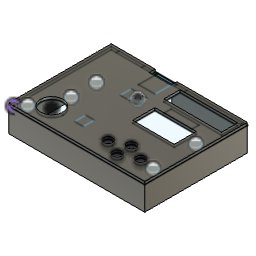
SmartDiskII Case v18 (Autodesk Fusion 360 design; units mm, degrees)
Autodesk Fusion 360 part; units mm, degrees
note: some values were not read from the file. Chosen so that the rebuilt part matches the saved one: which bodies a step acts on; which face or edge a step refers to. Set by a fixed rule: which sketch regions a step uses.
sketch "Sketch1" plane through (0, 0, 0) normal (0, 0, 1) x (1, 0, 0)
  line L0 (0, 0) -> (76.3, 0)
  line L1 (76.3, 0) -> (76.3, 56.8)
  line L2 (76.3, 56.8) -> (0, 56.8)
  line L3 (0, 56.8) -> (0, 0)
  line L4 (77.8, 58.3) -> (-1.5, 58.3)
  line L5 (-1.5, 58.3) -> (-1.5, -1.5)
  line L6 (-1.5, -1.5) -> (77.8, -1.5)
  line L7 (77.8, -1.5) -> (77.8, 58.3)
  line L8 (2.9, 56.8) -> (2.9, 58.3)
  line L9 (17.8, 56.8) -> (17.8, 58.3)
  line L10 (25.6, 56.8) -> (25.6, 58.3)
  line L11 (35.2, 58.3) -> (35.2, 56.8)
  line L12 (75.3, 58.3) -> (75.3, 56.8)
  line L13 (42.6, 58.3) -> (42.6, 56.8)
  line L14 (43.4, 38.8) -> (67.6, 38.8)
  line L15 (67.6, 38.8) -> (67.6, 25.9)
  line L16 (67.6, 25.9) -> (43.4, 25.9)
  line L17 (43.4, 25.9) -> (43.4, 38.8)
  circle A0 centre (65.2, 8.8) radius 2.5
  circle A1 centre (46.2, 8.8) radius 2.5
  circle A2 centre (55.6, 4.6) radius 2.5
  circle A3 centre (55.6, 12.9) radius 2.5
  line L18 (41.7, 55.2) -> (75.3, 55.2)
  line L19 (75.3, 55.2) -> (75.3, 45.8)
  line L20 (75.3, 45.8) -> (41.7, 45.8)
  line L21 (41.7, 45.8) -> (41.7, 55.2)
  line L22 (25.6, 56.8) -> (35.2, 56.8)
  line L23 (35.2, 56.8) -> (35.2, 47.1)
  line L24 (35.2, 47.1) -> (25.6, 47.1)
  line L25 (25.6, 47.1) -> (25.6, 56.8)
  line L26 (25.6, 42.9) -> (35.2, 42.9)
  line L27 (35.2, 42.9) -> (35.2, 36.4)
  line L28 (35.2, 36.4) -> (25.6, 36.4)
  line L29 (25.6, 36.4) -> (25.6, 42.9)
  circle A4 centre (12.4, 9.7) radius 6.5
  line L30 (25.6, 16.35) -> (30.6, 16.35)
  line L31 (30.6, 16.35) -> (30.6, 9.85)
  line L32 (30.6, 9.85) -> (25.6, 9.85)
  line L33 (25.6, 9.85) -> (25.6, 16.35)
  circle A5 centre (12.4, 21) radius 2.5
  circle A6 centre (12.4, 35.8) radius 2.5
  circle A7 centre (72.3819, 33.8) radius 2.5
  circle A8 centre (3.8963, 4.2747) radius 2.5
  circle A9 centre (72.3819, 8.8) radius 2.5
  line L34 (47.4, 40.3) -> (63.6, 40.3)
  line L35 (63.6, 40.3) -> (63.6, 44.3)
  line L36 (63.6, 44.3) -> (47.4, 44.3)
  line L37 (47.4, 44.3) -> (47.4, 40.3)
  line L38 (24.1, 58.3) -> (36.7, 58.3)
  line L39 (36.7, 58.3) -> (36.7, 56.8)
  line L40 (36.7, 56.8) -> (24.1, 56.8)
  line L41 (24.1, 56.8) -> (24.1, 58.3)
  line L42 (30.1, 42.9) -> (30.1, 36.4)
  line L43 (30.1, 36.4) -> (35.2, 42.9) construction
  line L44 (30.1, 42.9) -> (35.2, 36.4) construction
  circle A10 centre (32.65, 39.65) radius 2
  dimension "d5" = 76.3
  dimension "d6" = 56.8
  dimension "d8" = 1.5
  dimension "d9" = 2.9
  dimension "d10" = 17.8
  dimension "d11" = 25.6
  dimension "d12" = 35.2
  dimension "d13" = 75.3
  dimension "d14" = 42.6
  dimension "d15" = 8.7
  dimension "d16" = 24.2
  dimension "d17" = 12.9
  dimension "d18" = 25.9
  dimension "d19" = 5
  dimension "d20" = 8.8
  dimension "d21" = 11.1
  dimension "d22" = 5
  dimension "d23" = 30.1
  dimension "d24" = 5
  dimension "d25" = 4.6
  dimension "d26" = 20.7
  dimension "d27" = 5
  dimension "d28" = 12.9
  dimension "d39" = 9.4
  dimension "d40" = 1.6
  dimension "d43" = 8.8
  dimension "d44" = 1
  dimension "d45" = 33.6
  dimension "d46" = 20.7
  dimension "d47" = 9.7
  dimension "d48" = 6.5
  dimension "d50" = 13.9
  dimension "d53" = 13
  dimension "d54" = 12.4
  dimension "d55" = 9.7
  dimension "d58" = 9.85
  dimension "d59" = 6.5
  dimension "d60" = 5
  dimension "d67" = 5
  dimension "d68" = 5
  dimension "d69" = 21
  dimension "d70" = 21
  dimension "d71" = 5
  dimension "d72" = 5
  dimension "d73" = 23
  dimension "d74" = 5
  dimension "d86" = 4
  dimension "d87" = 4
  dimension "d88" = 1.5
  dimension "d89" = 1.5
  dimension "d92" = 12.6
  dimension "d93" = 1.5
  dimension "d94" = 1.5
  dimension "d113" = 4.5
  dimension "d135" = 4
  constraint horizontal L0
  constraint vertical L1
  constraint horizontal L2
  constraint vertical L3
  constraint coincident L0.start L3.end
  constraint coincident L2 L8.start
  constraint coincident L4 L8.end
  constraint perpendicular L4 L8
  constraint coincident L2 L9.start
  constraint coincident L4 L9.end
  constraint perpendicular L4 L9
  constraint coincident L2 L10.start
  constraint coincident L4 L10.end
  constraint perpendicular L4 L10
  constraint coincident L4 L11.start
  constraint coincident L2 L11.end
  constraint perpendicular L2 L11
  constraint coincident L4 L12.start
  constraint coincident L2 L12.end
  constraint perpendicular L2 L12
  constraint coincident L4 L13.start
  constraint coincident L2 L13.end
  constraint perpendicular L2 L13
  constraint horizontal L14
  constraint vertical L15
  constraint horizontal L16
  constraint vertical L17
  constraint horizontal L18
  constraint vertical L19
  constraint horizontal L20
  constraint vertical L21
  constraint horizontal L22
  constraint vertical L23
  constraint horizontal L24
  constraint vertical L25
  constraint horizontal L26
  constraint vertical L27
  constraint horizontal L28
  constraint vertical L29
  constraint horizontal L30
  constraint vertical L31
  constraint horizontal L32
  constraint vertical L33
  constraint collinear L29 L33
  constraint horizontal L34
  constraint vertical L35
  constraint horizontal L36
  constraint vertical L37
  constraint horizontal L38
  constraint vertical L39
  constraint horizontal L40
  constraint vertical L41
  constraint coincident L4 L38.start
  constraint coincident L26 L42.start
  constraint coincident L28 L42.end
  constraint perpendicular L28 L42
  constraint midpoint L44 A10.centre
  measures "d5" distance of L0.start L0.end
  measures "d6" distance of L0.start L2.end
  measures "d9" distance of L3 L8
  measures "d10" distance of L3 L9
  measures "d11" distance of L3 L10
  measures "d12" distance of L3 L11
  measures "d13" distance of L3 L12
  measures "d14" distance of L3 L13
  measures "d15" distance of L1 L15
  measures "d16" distance of L15 L17
  measures "d17" distance of L14 L16
  measures "d18" distance of L0 L16
  measures "d19" diameter of A0
  measures "d20" distance of L0 A0.centre
  measures "d21" distance of L1 A0.centre
  measures "d22" diameter of A1
  measures "d23" distance of L1 A1.centre
  measures "d24" diameter of A2
  measures "d25" distance of L0 A2.centre
  measures "d26" distance of L1 A2.centre
  measures "d27" diameter of A3
  measures "d28" distance of L0 A3.centre
  measures "d39" distance of L18.start L20.end
  measures "d40" distance of L2 L18
  measures "d43" distance of L0 A1.centre
  measures "d44" distance of L1 L19
  measures "d45" distance of L19 L21
  measures "d46" distance of L1 A3.centre
  measures "d47" distance of L10.start L24.end
  measures "d48" distance of L26.start L28.end
  measures "d50" distance of L2 L26
  measures "d53" diameter of A4
  measures "d54" distance of L3 A4.centre
  measures "d55" distance of L0 A4.centre
  measures "d58" distance of L0 L32
  measures "d59" distance of L30 L32
  measures "d60" distance of L31 L33
  measures "d67" diameter of A5
  measures "d68" diameter of A6
  measures "d69" distance of L2 A6.centre
  measures "d70" distance of L0 A5.centre
  measures "d71" diameter of A7
  measures "d72" diameter of A8
  measures "d73" distance of L2 A7.centre
  measures "d74" diameter of A9
  measures "d86" distance of L17 L37
  measures "d87" distance of L15 L35
  measures "d88" distance of L20 L36
  measures "d89" distance of L14 L34
  measures "d92" distance of L38.start L38.end
  measures "d93" distance of L10 L41
  measures "d94" distance of L11 L39
  measures "d113" distance of L29 L42
  measures "d135" diameter of A10
extrude "Extrude1" add sketch "Sketch1" along normal blind 1.5 contours L0 L1 L2 L3 L23 L24 L25 L40 | L2 L22 L23 L24 L25 L40 | L18 L19 L20 L21 | L26 L28 L29 L42 | L26 L27 L28 L42 | A4 | L30 L31 L32 L33 | A5 | A6 | A7 | A8 | A9 | L34 L35 L36 L37 | A10 makes body 1
extrude "Extrude2" add sketch "Sketch1" against normal blind 10 contours L0 L1 L2 L3 L4 L5 L6 L7 L8 L12 | L2 L4 L12 L13 | L2 L4 L9 L41 | L2 L4 L13 L39 | L2 L4 L10 L38 L40 L41 | L2 L4 L11 L38 L39 L40 bodies 1
extrude "Extrude3" add sketch "Sketch1" along normal blind 1.5 separate body contours L0 L1 L2 L3 L4 L5 L6 L7 L8 L12 | L2 L4 L8 L9 | L2 L4 L12 L13 | L2 L4 L9 L41 | L2 L4 L13 L39 | L2 L4 L10 L38 L40 L41 | L2 L4 L11 L38 L39 L40 | L2 L4 L10 L11 L22 L38 L40 makes body 2
extrude "Extrude4" cut sketch "Sketch1" along normal blind 1.5 contours L18 L19 L20 L21 bodies 1
extrude "Extrude5" cut sketch "Sketch1" along normal blind 3 contours L2 L4 L10 L11 L22 L38 L40 | L2 L22 L23 L24 L25 L40 | L26 L28 L29 L42 | L26 L27 L28 L42 | A4 | L30 L31 L32 L33 | A10 bodies 1 2
sketch "Sketch2" plane through (0, 0, 0) normal (0, 0, 1) x (1, 0, 0)
  circle A0 centre (55.6, 12.9) radius 2.25
  circle A1 centre (55.6, 12.9) radius 3.25
  line L0 (1.5, 1.5) -> (74.8, 1.5)
  line L1 (74.8, 1.5) -> (74.8, 55.3)
  line L2 (74.8, 55.3) -> (1.5, 55.3)
  line L3 (1.5, 55.3) -> (1.5, 1.5)
  line L4 (0, 56.8) -> (0, 0)
  line L5 (0, 0) -> (76.3, 0)
  line L6 (76.3, 0) -> (76.3, 56.8)
  line L7 (76.3, 56.8) -> (0, 56.8)
  line L8 (76.2, 0.1) -> (0.1, 0.1)
  line L9 (0.1, 0.1) -> (0.1, 56.7)
  line L10 (0.1, 56.7) -> (76.2, 56.7)
  line L11 (76.2, 56.7) -> (76.2, 0.1)
  circle A2 centre (32.65, 39.65) radius 2.5
  circle A3 centre (32.65, 39.65) radius 1.75
  point P0 (55.6, 12.9)
  point P1 (32.65, 39.65)
  dimension "d61" = 4.5
  dimension "d62" = 6.5
  dimension "d101" = 1.5
  dimension "d102" = 1.5
  dimension "d103" = 1.5
  dimension "d104" = 1.5
  dimension "d121" = 0.1
  dimension "d122" = 0.1
  dimension "d123" = 0.1
  dimension "d124" = 0.1
  dimension "d136" = 5
  dimension "d137" = 3.5
  constraint coincident P0 A0.centre
  constraint horizontal L0
  constraint vertical L1
  constraint horizontal L2
  constraint vertical L3
  constraint horizontal L8
  constraint vertical L9
  constraint horizontal L10
  constraint vertical L11
  constraint coincident P1 A2.centre
  constraint concentric A2 A3
  measures "d61" diameter of A0
  measures "d62" diameter of A1
  measures "d101" distance of L3 L4
  measures "d102" distance of L0 L5
  measures "d103" distance of L1 L6
  measures "d104" distance of L2 L7
  measures "d121" distance of L7 L10
  measures "d122" distance of L6 L11
  measures "d123" distance of L5 L8
  measures "d124" distance of L4 L9
  measures "d136" diameter of A2
  measures "d137" diameter of A3
extrude "Extrude7" add sketch "Sketch2" along normal blind 1.7 separate body contours A1 makes body 3
extrude "Extrude8" add sketch "Sketch2" along normal blind 4 contours A0 bodies 3
extrude "Extrude9" add sketch "Sketch1" against normal blind 6.9 separate body contours A5 | A6 | A7 | A8 | A9 makes body 4 at (6.3932, 4.15, -4.6) makes body 5 at (14.8969, 35.6754, -4.6) makes body 6 at (74.8788, 33.6754, -4.6) makes body 7 at (14.8969, 20.8754, -4.6) makes body 8 at (74.8788, 8.6754, -4.6)
combine "Combine1" operation add target body 4 tool bodies 7 5 6 8 makes body 9 at (14.8969, 20.8754, -4.6) makes body 10 at (74.8788, 33.6754, -4.6) makes body 11 at (14.8969, 35.6754, -4.6) makes body 12 at (74.8788, 8.6754, -4.6)
extrude "Extrude10" add sketch "Sketch1" against normal blind 5 contours L2 L4 L8 L9 bodies 1 3 2
extrude "Extrude11" add 2 faces at (25.4333, -1, -10) (23, 57.3, -10) along direction (0, 0, -1) blind 4 on bodies 1 bodies 1
extrude "Extrude12" add sketch "Sketch1" along normal blind 0.75 from surface at 0.75 contours L2 L22 L23 L24 L25 L40 | L30 L31 L32 L33 bodies 1
extrude "Extrude13" cut 1 faces at (32, 56.8, 1) along direction (0, -1, 0) blind 2 on bodies 1 bodies 1
extrude "Extrude14" cut sketch "Sketch1" along normal blind 0.75 contours L34 L35 L36 L37 bodies 1
extrude "Extrude15" cut sketch "Sketch1" along normal blind 1.5 contours L2 L4 L10 L38 L40 L41 | L2 L4 L11 L38 L39 L40 bodies 1
extrude "Extrude16" cut 2 faces at (36.2, 56.8, 0.5) (25.1, 56.8, 1) along direction (0, 1, 0) up to surface end surface through (35.2, 54.8, 0.75) normal (0, 1, 0) offset 0 on bodies 1 bodies 1
extrude "Extrude17" cut sketch "Sketch1" against normal blind 4 contours L2 L4 L10 L38 L40 L41 | L2 L4 L11 L38 L39 L40 bodies 1
fillet "Fillet1" radius 2 1 edges at (24.1, 57.55, -4) on bodies 1
fillet "Fillet1" radius 2 1 edges at (36.7, 57.55, -4) on bodies 1
extrude "Extrude18" add sketch "Sketch1" sketch "Sketch2" along normal blind 1.5 separate body contours L0 L1 L2 L3 L4 L5 L6 L7 L8 L12 | L2 L4 L8 L9 | L2 L4 L12 L13 | L2 L4 L9 L41 | L2 L4 L13 L39 | L2 L4 L10 L38 L40 L41 | L2 L4 L11 L38 L39 L40 | L2 L4 L10 L11 L22 L38 L40 of sketch 2 contours A0 | A1 | L0 L1 L2 L3 | L4 L5 L6 L7 | L8 L9 L10 L11 | A2 | A3 makes body 13
extrude "Extrude19" add sketch "Sketch2" along normal blind 6.7 contours L8 L9 L10 L11 bodies 13
extrude "Extrude20" add sketch "Sketch1" along normal blind 8.6 contours L2 L4 L8 L9 bodies 13
extrude "Extrude21" add sketch "Sketch1" along normal blind 9.5 contours L2 L4 L10 L11 L22 L38 L40 bodies 13
extrude "Extrude22" add sketch "Sketch1" along normal blind 0.75 from surface at 0.75 contours L26 L28 L29 L42 bodies 1
extrude "Extrude23" add 1 faces at (28.8, 57.8, 9.5) along direction (0, 0, 1) blind 2 on bodies 13 bodies 13
extrude "Extrude24" cut 1 faces at (25.6, 57.8, 8.1667) along direction (1, 0, 0) blind 0.1 on bodies 13 bodies 13
extrude "Extrude25" cut 1 faces at (2.9, 57.8, 6.2333) along direction (1, 0, 0) blind 0.1 on bodies 13 bodies 13
extrude "Extrude26" cut 1 faces at (17.8, 57.8, 6.2333) along direction (-1, 0, 0) blind 0.1 on bodies 13 bodies 13
extrude "Extrude27" cut 1 faces at (35.2, 57.8, 4.8333) along direction (-1, 0, 0) blind 0.1 on bodies 13 bodies 13
extrude "Extrude28" add sketch "Sketch2" along normal blind 0.5 separate body contours A2 makes body 14
extrude "Extrude29" add sketch "Sketch2" along normal blind 1.75 contours A3 bodies 14
extrude "Extrude30" add sketch "Sketch1" along normal blind 0.75 from surface at 0.75 contours L26 L27 L28 L42 bodies 1
hidden bodies 3 4 9 10 11 12 13 14
equation "width = 76 mm"
equation "length = 56.5 mm"
equation "margin = 0.3 mm"
equation "d5 = width + margin"
equation "d6 = length + margin"
equation "wall_ep = 1.5 mm"
equation "d8 = wall_ep"
equation "d9 = margin + 2.6 mm"
equation "d10 = margin + 17.5 mm"
equation "d11 = margin + 25.3 mm"
equation "d12 = margin + 34.90 mm"
equation "d13 = margin + 75 mm"
equation "d14 = margin + 42.30 mm"
equation "d33 = wall_ep"
equation "d37 = wall_ep"
equation "d39 = 8.8 mm + 0.6 mm"
equation "d40 = 1.9 mm - 0.3 mm"
equation "d41 = wall_ep"
equation "d45 = 33.10 mm + 0.5 mm"
equation "d77 = -5.6 mm + 1.5 mm - 0.9 mm"
equation "d101 = wall_ep"
equation "d102 = wall_ep"
equation "d103 = wall_ep"
equation "d104 = wall_ep"
equation "d107 = 1.5 mm + 5.2 mm"
equation "d109 = 1.5 mm + 7.1 mm"
equation "d111 = 8 mm + 1.5 mm"
named bodies: "bouton", "couvercle", "bouton RESET"
